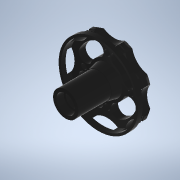
# Autodesk Inventor part: BASE
Saved by Autodesk Inventor 2022 (Build 260153000, 153)
## iProperties
Created: 2022-07-26
Part Number: BASE
Material: Stainless Steel
Document SubType Name: Modeling
Designer: Nathan Cai
Density: 8 g/cm^3
Appearance: Smooth - Black
Author: Nathan Cai
Autodesk Inventor part; units mm, degrees
ref_plane "YZ Plane" through (0, 0, 0) normal (1, 0, 0) x (0, 1, 0)
ref_plane "XZ Plane" through (0, 0, 0) normal (0, 1, 0) x (-1, 0, 0)
ref_plane "XY Plane" through (0, 0, 0) normal (0, 0, 1) x (1, 0, 0)
sketch "Sketch1" plane through (0, 0, 0) normal (0, 1, 0) x (-1, 0, 0)
  line L0 (0, 0) -> (21.25, 0)
  line L1 (21.25, 0) -> (21.25, -6.5)
  line L2 (21.25, -6.5) -> (0, -6.5) construction
  line L3 (0, -6.5) -> (0, 0)
  line L4 (0, -6.5) -> (20, -6.5) construction
  line L5 (20, -6.5) -> (20, -8.5) construction
  line L6 (20, -8.5) -> (0, -8.5)
  line L7 (0, -8.5) -> (0, -6.5)
  line L8 (21.25, -6.5) -> (20, -8.5)
  line L9 (21.25, -1.6) -> (20.75, -1.6)
  line L10 (20.75, -1.6) -> (20.75, -2.6)
  line L11 (20.75, -2.6) -> (21.25, -2.6) construction
  line L12 (21.25, -2.6) -> (21.25, -1.6)
  line L13 (21.25, -3.4) -> (20.75, -3.4)
  line L14 (20.75, -3.4) -> (20.75, -4.4)
  line L15 (20.75, -4.4) -> (21.25, -4.4)
  line L16 (21.25, -4.4) -> (21.25, -3.4)
  line L17 (0, 0) -> (20, 0) construction
  line L18 (20, 0) -> (20, -4.75)
  line L19 (20, -4.75) -> (5, -4.75)
  line L20 (0, -4.75) -> (0, 0)
  line L21 (5, -4.75) -> (8, -4.75)
  line L22 (8, -4.75) -> (8, 0) construction
  line L23 (8, 0) -> (0, 0)
  line L24 (0, 0) -> (0, -4.75)
  line L25 (8, -4.75) -> (7, 0)
  line L26 (0, -8.5) -> (5, -8.5)
  line L27 (5, -8.5) -> (5, -4.5)
  line L28 (5, -4.5) -> (0, -4.5)
  line L29 (0, -4.5) -> (0, -8.5)
  line L30 (0, -4.5) -> (4, -4.5)
  line L31 (4, -4.5) -> (4, 13.5)
  line L32 (4, 13.5) -> (0, 13.5)
  line L33 (0, 13.5) -> (0, -4.5)
  line L34 (0, 13.5) -> (5, 13.5)
  line L35 (5, 13.5) -> (5, 17.5)
  line L36 (5, 17.5) -> (0, 17.5)
  line L37 (0, 17.5) -> (0, 13.5)
  line L38 (0, 17.5) -> (6.75, 17.5)
  line L39 (6.75, 17.5) -> (6.75, 0)
  line L40 (6.75, 0) -> (0, 0)
  line L41 (0, 0) -> (0, 17.5)
  point P0 (6.75, 0)
  dimension "d0" = 21.25
  dimension "d1" = 6.5
  dimension "d2" = 20
  dimension "d3" = 2
  dimension "d4" = 1.6
  dimension "d5" = 1
  dimension "d6" = 1
  dimension "d7" = 0.8
  dimension "d8" = 0.5
  dimension "d9" = 1.25
  dimension "d10" = 3.75
  dimension "d11" = 8
  dimension "d12" = 7
  dimension "d13" = 5
  dimension "d14" = 4
  dimension "d15" = 4
  dimension "d16" = 18
  dimension "d17" = 5
  dimension "d18" = 4
  dimension "d19" = 6.75
  constraints: 84 end point, 20 parallel, 10 horizontal, 10 perpendicular, 7 point on line
  measures "d0" distance of L1.end L2.end
  measures "d1" distance of L0.end L1.end
  measures "d2" distance of L5.end L6.end
  measures "d3" distance of L4.end L5.end
  measures "d4" distance between parallel lines of L0 L9
  measures "d5" distance of L9.end L10.end
  measures "d6" distance of L13.end L14.end
  measures "d7" distance between parallel lines of L11 L13
  measures "d8" distance between parallel lines of L12 L10
  measures "d9" distance between parallel lines of L1 L18
  measures "d10" distance between parallel lines of L6 L19
  measures "d11" distance of L23.end L22.end
  measures "d12" distance from line of L3 L25.end
  measures "d13" distance of L28.end L27.end
  measures "d14" distance of L27.end L26.end
  measures "d15" distance of L32.end L31.end
  measures "d16" distance of L31.end L30.end
  measures "d17" distance of L36.end L35.end
  measures "d18" distance of L35.end L34.end
  measures "d19" distance of L39.end L40.end
revolve "Revolution1" add sketch "Sketch1" angle 360 about axis through (0, 0, 13.5) along (0, 0, -1) contours L0 L25 L19 L27 L28 L31 | L0 L31 L34 L35 L38 L39 | L19 L18 L0 L1 L13 L14 L15 L8 L6 L27
sketch "Sketch2" plane through (0, 0, -8.5) normal (0, 0, -1) x (-1, 0, 0)
  circle A0 centre (0, 0) radius 12.5 construction
  circle A1 centre (0, 12.5) radius 1.5
  line L0 (0, 17.5) -> (0, 0) construction
  arc A2 (11.782, 5.494) -> (5.494, 11.782) centre (0, 0) ccw construction
  arc A3 (14.9541, 6.9732) -> (6.9732, 14.9541) centre (0, 0) ccw
  arc A4 (8.6099, 4.0149) -> (4.0149, 8.6099) centre (0, 0) ccw
  arc A5 (8.6099, 4.0149) -> (14.9541, 6.9732) centre (11.782, 5.494) ccw
  arc A6 (6.9732, 14.9541) -> (4.0149, 8.6099) centre (5.494, 11.782) ccw
  line L1 (5.494, 11.782) -> (0, 0) construction
  line L2 (0, 0) -> (11.782, 5.494) construction
  circle A7 centre (0, 0) radius 17.5 construction
  circle A8 centre (0, 27.5) radius 10
  circle A9 centre (-12.5, 0) radius 1.5
  arc A10 (-14.9541, 6.9732) -> (-8.6099, 4.0149) centre (-11.782, 5.494) ccw
  arc A11 (-4.0149, 8.6099) -> (-8.6099, 4.0149) centre (0, 0) ccw
  arc A12 (-6.9732, 14.9541) -> (-14.9541, 6.9732) centre (0, 0) ccw
  arc A13 (-4.0149, 8.6099) -> (-6.9732, 14.9541) centre (-5.494, 11.782) ccw
  circle A14 centre (0, -12.5) radius 1.5
  arc A15 (-6.9732, -14.9541) -> (-4.0149, -8.6099) centre (-5.494, -11.782) ccw
  arc A16 (-8.6099, -4.0149) -> (-4.0149, -8.6099) centre (0, 0) ccw
  arc A17 (-14.9541, -6.9732) -> (-6.9732, -14.9541) centre (0, 0) ccw
  arc A18 (-8.6099, -4.0149) -> (-14.9541, -6.9732) centre (-11.782, -5.494) ccw
  circle A19 centre (12.5, 0) radius 1.5
  arc A20 (14.9541, -6.9732) -> (8.6099, -4.0149) centre (11.782, -5.494) ccw
  arc A21 (4.0149, -8.6099) -> (8.6099, -4.0149) centre (0, 0) ccw
  arc A22 (6.9732, -14.9541) -> (14.9541, -6.9732) centre (0, 0) ccw
  arc A23 (4.0149, -8.6099) -> (6.9732, -14.9541) centre (5.494, -11.782) ccw
  circle A24 centre (-19.4454, 19.4454) radius 10
  circle A25 centre (-27.5, 0) radius 10
  circle A26 centre (-19.4454, -19.4454) radius 10
  circle A27 centre (0, -27.5) radius 10
  circle A28 centre (19.4454, -19.4454) radius 10
  circle A29 centre (27.5, 0) radius 10
  circle A30 centre (19.4454, 19.4454) radius 10
  point P0 (-12.3744, 12.3744)
  point P1 (-17.5, 0)
  point P2 (-12.3744, -12.3744)
  point P3 (0, -17.5)
  point P4 (12.3744, -12.3744)
  point P5 (17.5, 0)
  point P6 (12.3744, 12.3744)
  dimension "d21" = 25
  dimension "d27" = 20
  dimension "d22" = 3
  dimension "d23" = 7
  dimension "d24" = 25
  dimension "d25" = 0.5
  dimension "d26" = 40
  dimension "d28" = 35
  dimension "d31" = 360
  dimension "d35" = 360
  constraints: 34 point on circle, 22 centre point, 6 end point, 4 tangent, 3 coincident, 3 vertical alignment, 2 horizontal alignment, 2 point on line, 1 vertical, 101 other
  measures "d22" diameter of A1
  measures "d23" diameter of A5
  measures "d24" angle of L0 L1
  measures "d26" angle of L1 L2
  measures "d28" diameter of A7
extrude "Extrusion1" cut sketch "Sketch2" against normal blind 6
body "Solid1"
